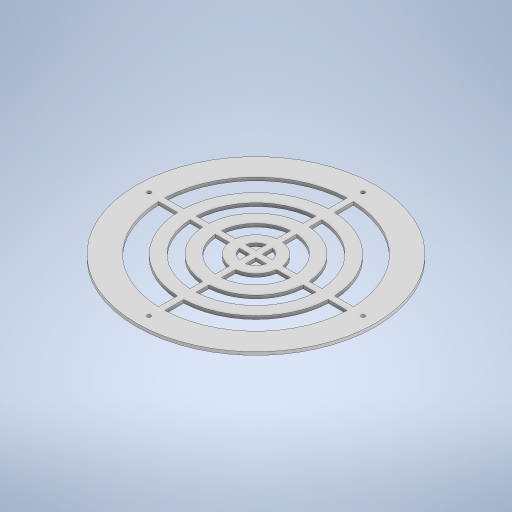
# Autodesk Inventor part: Part1
Saved by Autodesk Inventor 2024 (Build 280153000, 153)
## iProperties
Created: 2023-10-29
Part Number: Part1
Material: Generic
Document SubType Name: Modeling
Designer: felip
Density: 1 g/cm^3
Appearance: Default
Author: felip
Autodesk Inventor part; units mm, degrees
ref_plane "YZ Plane" through (0, 0, 0) normal (1, 0, 0) x (0, 1, 0)
ref_plane "XZ Plane" through (0, 0, 0) normal (0, 1, 0) x (-1, 0, 0)
ref_plane "XY Plane" through (0, 0, 0) normal (0, 0, 1) x (1, 0, 0)
sketch "Sketch1" plane through (0, 0, 0) normal (0, 1, 0) x (-1, 0, 0)
  circle A0 centre (0, 0) radius 95
  circle A1 centre (85, 0) radius 1.5
  circle A2 centre (0, 85) radius 1.5
  circle A3 centre (-85, 0) radius 1.5
  circle A4 centre (0, -85) radius 1.5
  line L0 (-2.5, -74.9583) -> (2.5, 74.9583) construction
  arc A5 (-8.8904, -12.0814) -> (-9.3573, -11.7235) centre (0, 0) ccw construction
  arc A6 (-22.389, -26.9023) -> (-22.6552, -26.6785) centre (0, 0) ccw construction
  line L1 (-2.5, 74.9583) -> (-2.5, 59.9479)
  line L2 (2.5, 59.9479) -> (2.5, 74.9583)
  line L3 (0, 74.9583) -> (0, 75)
  line L4 (-2.5, 49.9375) -> (-2.5, 39.9218)
  line L5 (2.5, 39.9218) -> (2.5, 49.9375)
  line L6 (2.5, 18.8348) -> (2.5, 29.8957)
  line L7 (-2.5, 29.8957) -> (-2.5, 18.8348)
  arc A7 (-35.5953, -41.9282) -> (-55, 0) centre (0, 0) ccw construction
  arc A8 (-54.9694, -1.8333) -> (-36.2318, -41.3794) centre (0, 0) ccw construction
  line L8 (74.9583, -2.5) -> (-39.9778, 1.3333) construction
  line L9 (-54.9694, 1.8333) -> (-59.9667, 2) construction
  line L10 (-74.9583, -2.5) -> (-54.9694, -1.8333) construction
  line L11 (2.5, -74.9583) -> (-0.0834, 2.5) construction
  line L12 (-0.3667, 10.9939) -> (-0.5, 14.9917) construction
  arc A9 (-6.5196, -8.8597) -> (-6.6969, -8.7365) centre (-8.8904, -12.0814) ccw
  arc A10 (-11.5507, -15.0685) -> (-11.2612, -15.3031) centre (-8.8904, -12.0814) ccw
  arc A11 (-11.8525, -14.8498) -> (-11.5507, -15.0685) centre (-9.3573, -11.7235) ccw
  arc A12 (-6.6969, -8.7365) -> (-6.862, -8.5973) centre (-9.3573, -11.7235) ccw
  arc A13 (-19.1906, -23.0591) -> (-19.3066, -22.9655) centre (-22.389, -26.9023) ccw
  arc A14 (-25.7376, -30.6153) -> (-25.5875, -30.7454) centre (-22.389, -26.9023) ccw
  arc A15 (-25.8916, -30.4897) -> (-25.7376, -30.6153) centre (-22.6552, -26.6785) ccw
  arc A16 (-19.3066, -22.9655) -> (-19.4187, -22.8673) centre (-22.6552, -26.6785) ccw
  arc A17 (-32.3594, -38.1165) -> (-32.6602, -37.8804) centre (-35.5953, -41.9282) ccw
  arc A18 (-39.167, -45.4272) -> (-38.8313, -45.7398) centre (-35.5953, -41.9282) ccw
  arc A19 (-39.5256, -45.1412) -> (-39.167, -45.4272) centre (-36.2318, -41.3794) ccw
  arc A20 (-32.6602, -37.8804) -> (-32.938, -37.6176) centre (-36.2318, -41.3794) ccw
  line L13 (-0.6333, 18.9894) -> (-1.1667, 34.9806) construction
  line L14 (-1.3333, 39.9778) -> (-2.5, 74.9583) construction
  arc A21 (-2.5, 74.9583) -> (-74.9583, 2.5) centre (0, 0) ccw
  line L15 (-74.9583, 0) -> (-75, 0)
  arc A22 (-2.5, 59.9479) -> (-59.9479, 2.5) centre (0, 0) ccw
  arc A23 (-59.9479, -2.5) -> (-39.5256, -45.1412) centre (0, 0) ccw
  arc A24 (-2.5, 49.9375) -> (-49.9375, 2.5) centre (0, 0) ccw
  arc A25 (-49.9375, -2.5) -> (-32.938, -37.6176) centre (0, 0) ccw
  arc A26 (-39.9218, -2.5) -> (-25.8916, -30.4897) centre (0, 0) ccw
  arc A27 (-29.8957, -2.5) -> (-19.4187, -22.8673) centre (0, 0) ccw
  arc A28 (-2.5, 29.8957) -> (-29.8957, 2.5) centre (0, 0) ccw
  arc A29 (-2.5, 39.9218) -> (-39.9218, 2.5) centre (0, 0) ccw
  arc A30 (-18.8348, -2.5) -> (-11.8525, -14.8498) centre (0, 0) ccw
  arc A31 (-2.5, 18.8348) -> (-18.8348, 2.5) centre (0, 0) ccw
  arc A32 (-10.7121, -2.5) -> (-6.862, -8.5973) centre (0, 0) ccw
  arc A33 (-2.5, 10.7121) -> (-10.7121, 2.5) centre (0, 0) ccw
  line L16 (-2.5, 10.7121) -> (-2.5, 2.5)
  line L17 (-2.5, 0.0834) -> (-2.5, -0.0834)
  line L18 (-74.9583, -2.5) -> (-59.9479, -2.5)
  line L19 (-59.9479, 2.5) -> (-74.9583, 2.5)
  line L20 (-39.9218, 2.5) -> (-49.9375, 2.5)
  line L21 (-49.9375, -2.5) -> (-39.9218, -2.5)
  line L22 (-2.5, 2.5) -> (-10.7121, 2.5)
  line L23 (-18.8348, 2.5) -> (-29.8957, 2.5)
  line L24 (-29.8957, -2.5) -> (-18.8348, -2.5)
  line L25 (-10.7121, -2.5) -> (-2.5, -2.5)
  line L26 (-0.0834, -2.5) -> (0.0834, -2.5)
  line L27 (2.5, -0.0834) -> (2.5, 0.0834)
  line L28 (2.5, 2.5) -> (2.5, 10.7121)
  arc A34 (10.7121, 2.5) -> (2.5, 10.7121) centre (0, 0) ccw
  line L29 (2.5, -2.5) -> (10.7121, -2.5)
  line L30 (10.7121, 2.5) -> (2.5, 2.5)
  arc A35 (18.8348, 2.5) -> (2.5, 18.8348) centre (0, 0) ccw
  arc A36 (39.9218, 2.5) -> (2.5, 39.9218) centre (0, 0) ccw
  line L31 (74.9583, 0) -> (75, 0)
  arc A37 (29.8957, 2.5) -> (2.5, 29.8957) centre (0, 0) ccw
  line L32 (29.8957, 2.5) -> (18.8348, 2.5)
  line L33 (18.8348, -2.5) -> (29.8957, -2.5)
  arc A38 (49.9375, 2.5) -> (2.5, 49.9375) centre (0, 0) ccw
  line L34 (39.9218, -2.5) -> (49.9375, -2.5)
  line L35 (59.9479, -2.5) -> (74.9583, -2.5)
  line L36 (74.9583, 2.5) -> (59.9479, 2.5)
  line L37 (49.9375, 2.5) -> (39.9218, 2.5)
  arc A39 (59.9479, 2.5) -> (2.5, 59.9479) centre (0, 0) ccw
  line L38 (-49.9722, -1.6667) -> (54.9694, 1.8333) construction
  line L39 (59.9667, 2) -> (74.9583, 2.5) construction
  arc A40 (74.9583, 2.5) -> (2.5, 74.9583) centre (0, 0) ccw
  line L40 (74.9583, 0) -> (75, 0)
  line L41 (83.5, 0) -> (85, 0)
  arc A41 (-6.5196, -8.8597) -> (-2.5, -10.7121) centre (0, 0) ccw
  arc A42 (2.5, -10.7121) -> (10.7121, -2.5) centre (0, 0) ccw
  arc A43 (-11.2612, -15.3031) -> (-2.5, -18.8348) centre (0, 0) ccw
  arc A44 (2.5, -18.8348) -> (18.8348, -2.5) centre (0, 0) ccw
  line L42 (2.5, -10.7121) -> (2.5, -2.5)
  line L43 (-2.5, -2.5) -> (-2.5, -10.7121)
  arc A45 (-19.1906, -23.0591) -> (-2.5, -29.8957) centre (0, 0) ccw
  arc A46 (2.5, -29.8957) -> (29.8957, -2.5) centre (0, 0) ccw
  line L44 (2.5, -29.8957) -> (2.5, -18.8348)
  arc A47 (-25.5875, -30.7454) -> (-2.5, -39.9218) centre (0, 0) ccw
  arc A48 (2.5, -39.9218) -> (39.9218, -2.5) centre (0, 0) ccw
  line L45 (-2.5, -18.8348) -> (-2.5, -29.8957)
  arc A49 (-32.3594, -38.1165) -> (-2.5, -49.9375) centre (0, 0) ccw
  arc A50 (2.5, -49.9375) -> (49.9375, -2.5) centre (0, 0) ccw
  line L46 (2.5, -74.9583) -> (2.5, -59.9479)
  line L47 (2.5, -49.9375) -> (2.5, -39.9218)
  arc A51 (-38.8313, -45.7398) -> (-2.5, -59.9479) centre (0, 0) ccw
  arc A52 (2.5, -59.9479) -> (59.9479, -2.5) centre (0, 0) ccw
  line L48 (0, -74.9583) -> (0, -75)
  line L49 (-2.5, -39.9218) -> (-2.5, -49.9375)
  line L50 (-2.5, -59.9479) -> (-2.5, -74.9583)
  arc A53 (-74.9583, -2.5) -> (-2.5, -74.9583) centre (0, 0) ccw
  arc A54 (2.5, -74.9583) -> (74.9583, -2.5) centre (0, 0) ccw
  dimension "d2" = 3
  dimension "d0" = 190
  dimension "d1" = 85
  dimension "d5" = 360
  dimension "d8" = 5
  dimension "d9" = 15
  dimension "d11" = 35
  constraints: 153 parallel, 104 point on circle, 102 end point, 54 centre point, 11 horizontal, 9 point on line, 6 coincident, 1 horizontal alignment, 1 midpoint, 1 perpendicular, 11 other
  measures "d0" diameter of A0
  measures "d1" distance of A0.centre L41.end
  measures "d8" distance of L1.start L0.end
  measures "d9" radius of A5
  measures "d11" radius of A6
extrude "Extrusion1" add sketch "Sketch1" along normal blind 2.5
body "Solid1"
